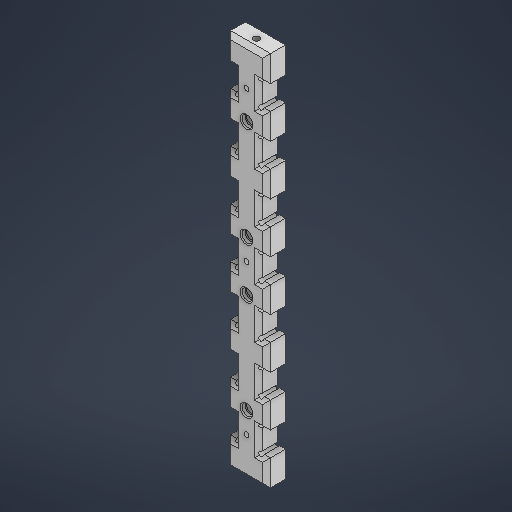
# Autodesk Inventor part: Locating_bar_V2_fit0
Saved by Autodesk Inventor 2026.1 (Build 301233020, 233B)
## iProperties
Created: 2023-09-05
Part Number: Locating_bar_V2_fit0
Material: Generic
Document SubType Name: Modeling
Designer: Joshua Harper
Density: 1 g/cm^3
Appearance: Default
Author: Joshua Harper
Autodesk Inventor part; units mm, degrees
ref_plane "YZ Plane" through (0, 0, 0) normal (1, 0, 0) x (0, 1, 0)
ref_plane "XZ Plane" through (0, 0, 0) normal (0, 1, 0) x (-1, 0, 0)
ref_plane "XY Plane" through (0, 0, 0) normal (0, 0, 1) x (1, 0, 0)
sketch "Sketch1" plane through (0, 0, 0) normal (0, 0, 1) x (1, 0, 0)
  line L0 (0, 94) -> (10, 94)
  line L1 (10, 94) -> (10, 81)
  line L2 (10, 81) -> (6, 81)
  line L3 (6, 81) -> (6, 69)
  line L4 (6, 69) -> (10, 69)
  line L5 (10, 69) -> (10, 56)
  line L6 (10, 56) -> (6, 56)
  line L7 (6, 56) -> (6, 44)
  line L8 (6, 44) -> (10, 44)
  line L9 (10, 44) -> (10, 31)
  line L10 (10, 31) -> (6, 31)
  line L11 (6, 31) -> (6, 19)
  line L12 (6, 19) -> (10, 19)
  line L13 (10, 19) -> (10, 6)
  line L14 (10, 6) -> (6, 6)
  line L15 (6, 6) -> (6, 0)
  line L16 (0, 0) -> (0, 65.9305) construction
  line L17 (0, 0) -> (38.6364, 0) construction
  line L18 (0, 94) -> (-10, 94)
  line L19 (-10, 94) -> (-10, 81)
  line L20 (-10, 81) -> (-6, 81)
  line L21 (-6, 81) -> (-6, 69)
  line L22 (-6, 69) -> (-10, 69)
  line L23 (-10, 69) -> (-10, 56)
  line L24 (-10, 56) -> (-6, 56)
  line L25 (-6, 56) -> (-6, 44)
  line L26 (-6, 44) -> (-10, 44)
  line L27 (-10, 44) -> (-10, 31)
  line L28 (-10, 31) -> (-6, 31)
  line L29 (-6, 31) -> (-6, 19)
  line L30 (-6, 19) -> (-10, 19)
  line L31 (-10, 19) -> (-10, 6)
  line L32 (-10, 6) -> (-6, 6)
  line L33 (-6, 6) -> (-6, 0)
  line L34 (0, 0) -> (-38.6364, 0) construction
  line L35 (0, -94) -> (10, -94)
  line L36 (10, -94) -> (10, -81)
  line L37 (10, -81) -> (6, -81)
  line L38 (6, -81) -> (6, -69)
  line L39 (6, -69) -> (10, -69)
  line L40 (10, -69) -> (10, -56)
  line L41 (10, -56) -> (6, -56)
  line L42 (6, -56) -> (6, -44)
  line L43 (6, -44) -> (10, -44)
  line L44 (10, -44) -> (10, -31)
  line L45 (10, -31) -> (6, -31)
  line L46 (6, -31) -> (6, -19)
  line L47 (6, -19) -> (10, -19)
  line L48 (10, -19) -> (10, -6)
  line L49 (10, -6) -> (6, -6)
  line L50 (6, -6) -> (6, 0)
  line L51 (0, 0) -> (0, -65.9305) construction
  line L52 (0, -94) -> (-10, -94)
  line L53 (-10, -94) -> (-10, -81)
  line L54 (-6, -69) -> (-10, -69)
  line L55 (-10, -81) -> (-6, -81)
  line L56 (-6, -81) -> (-6, -69)
  line L57 (-10, -69) -> (-10, -56)
  line L58 (-10, -56) -> (-6, -56)
  line L59 (-6, -56) -> (-6, -44)
  line L60 (-6, -44) -> (-10, -44)
  line L61 (-10, -44) -> (-10, -31)
  line L62 (-10, -31) -> (-6, -31)
  line L63 (-6, -31) -> (-6, -19)
  line L64 (-6, -19) -> (-10, -19)
  line L65 (-10, -19) -> (-10, -6)
  line L66 (-10, -6) -> (-6, -6)
  line L67 (-6, -6) -> (-6, 0)
  point P0 (6, 75)
  point P1 (5, 94)
  point P2 (-6, 75)
  point P3 (-5, 94)
  point P4 (6, -75)
  point P5 (5, -94)
  point P6 (-6, -75)
  point P7 (-5, -94)
  dimension "d0" = 10
  dimension "d1" = 13
  dimension "d2" = 12
  dimension "d3" = 6
  dimension "d4" = 6
  constraints: 136 end point, 55 symmetric about line, 44 point on line, 10 perpendicular, 6 collinear, 3 horizontal, 2 midpoint, 1 vertical
  measures "d0" distance of L0.start L0.end
  measures "d1" distance of L0.end L1.end
  measures "d2" distance between parallel lines of L4 L2
  measures "d3" distance from line of L16 point (6, 75)
  measures "d4" distance between parallel lines of L17 L14
extrude "Extrusion1" add sketch "Sketch1" along normal blind 9.5
chamfer "Chamfer1" distance 2 angle 45 64 edges at (-10, 87.5, 9.5) (10, 87.5, 9.5) (-8, 81, 9.5) (8, 81, 9.5) (6, 75, 9.5) (-6, 75, 9.5) (-8, 69, 9.5) (-10, 62.5, 9.5) (8, 69, 9.5) (10, 62.5, 9.5) (8, 56, 9.5) (-8, 56, 9.5) (6, 50, 9.5) (-6, 50, 9.5) (-8, 44, 9.5) (8, 44, 9.5) (10, 37.5, 9.5) (-10, 37.5, 9.5) (-8, 31, 9.5) (8, 31, 9.5) (6, 25, 9.5) (-6, 25, 9.5) (-8, 19, 9.5) (8, 19, 9.5) (10, 12.5, 9.5) (-10, 12.5, 9.5) (8, 6, 9.5) (-8, 6, 9.5) (-6, -3, 9.5) (-6, 3, 9.5) (6, 3, 9.5) (6, -3, 9.5) (8, -6, 9.5) (-8, -6, 9.5) (-10, -12.5, 9.5) (10, -12.5, 9.5) (8, -19, 9.5) (-8, -19, 9.5) (-6, -25, 9.5) (6, -25, 9.5) (8, -31, 9.5) (-8, -31, 9.5) (-10, -37.5, 9.5) (10, -37.5, 9.5) (-8, -44, 9.5) (8, -44, 9.5) (6, -50, 9.5) (-6, -50, 9.5) (-8, -56, 9.5) (8, -56, 9.5) (10, -62.5, 9.5) (-10, -62.5, 9.5) (8, -69, 9.5) (-8, -69, 9.5) (-6, -75, 9.5) (6, -75, 9.5) (8, -81, 9.5) (-8, -81, 9.5) (-10, -87.5, 9.5) (10, -87.5, 9.5) (5, -94, 9.5) (-5, -94, 9.5) (-5, 94, 9.5) (5, 94, 9.5)
sketch "Sketch2" plane through (-10, 94, 0) normal (0, 1, 0) x (1, 0, 0)
  line L0 (20, 0) -> (0, 0) projected
  line L1 (10, 0) -> (10, -4.5) construction
  line L2 (2, -9.5) -> (18, -9.5) projected
  dimension "d19" = 5
  constraints: 2 end point, 1 vertical
  measures "d19" distance from line of L2 L1.end
hole "Hole1" at (0, 94, 4.5) direction (0, -1, 0) diameter 3.242 depth 11.8 tip angle 118 thread size "M4x0.7" class "6H" standard "ANSI Metric M Profile"
mirror "Mirror1" about plane through (0, 0, 0) normal (0, 1, 0) of "Hole1"
sketch "Sketch3" plane through (0, 0, 0) normal (0, 0, -1) x (-1, 0, 0)
  line L0 (0, 0) -> (0, 75) construction
  line L1 (0, 0) -> (31.7018, 0) construction
  point P0 (0, -75)
  dimension "d28" = 75
  constraints: 4 end point, 1 coincident, 1 horizontal, 1 symmetric about line, 1 vertical
  measures "d28" distance of L0.end point (0, 0)
hole "Hole2" at (0, 0, 0) at (0, 75, 0) at (0, -75, 0) direction (0, 0, 1) diameter 2.459 end through all counterbore diameter 4 counterbore depth 2 thread size "M3x0.5" class "6H" standard "ANSI Metric M Profile"
sketch "Sketch4" plane through (0, 0, 0) normal (0, 0, -1) x (-1, 0, 0)
  circle A0 centre (0, 0) radius 1.2295 construction
  line L0 (0, 0) -> (0, -14.5) construction
  line L1 (15.0532, -2) -> (-13.6223, -2) construction
  point P0 (0, -64.5)
  point P1 (0, 10.5)
  point P2 (0, 60.5)
  dimension "d36" = 14.5
  dimension "d82" = 64.5
  dimension "d83" = 2
  constraints: 4 end point, 2 symmetric about line, 1 horizontal, 1 vertical
  measures "d36" distance of L0.end point (0, 0)
  measures "d82" distance of point (0, -64.5) point (0, 0)
  measures "d83" distance from line of L1 point (0, 0)
hole "Hole3" at (0, -14.5, 0) at (0, -64.5, 0) at (0, 10.5, 0) at (0, 60.5, 0) direction (0, 0, 1) diameter 4.5 end through all counterbore diameter 8 counterbore depth 3 clearance for "Slotted Cheese Head Screw DIN 84" size "M4" standard "DIN"
sketch "Sketch5" plane through (0, 0, 9.5) normal (0, 0, 1) x (1, 0, 0)
  line L0 (-10, -81) -> (-10, -94) construction
  line L1 (-10, -94) -> (10, -94) construction
  circle A0 centre (0, -14.5) radius 2.25 construction
  circle A1 centre (0, -14.5) radius 2.25 construction
  circle A2 centre (0, -64.5) radius 2.25 construction
  circle A3 centre (0, -64.5) radius 2.25 construction
  circle A4 centre (0, 0) radius 1.2295 construction
  circle A5 centre (0, 10.5) radius 2.25 construction
  circle A6 centre (0, 10.5) radius 2.25 construction
  circle A7 centre (0, 60.5) radius 2.25 construction
  circle A8 centre (0, 60.5) radius 2.25 construction
  circle A9 centre (0, 10.5) radius 2.25 projected
  circle A10 centre (0, 60.5) radius 2.25 projected
  constraints: 6 centre point, 6 coincident, 5 concentric, 1 vertical alignment
hole "Hole4" at (0, -64.5, 9.5) at (0, -14.5, 9.5) at (0, 60.5, 9.5) at (0, 10.5, 9.5) direction (0, 0, -1) diameter 5.5 depth 2 tip angle 118
chamfer "Chamfer2" distance 0.5 angle 45 4 edges at (0, -61.75, 9.5) (0, -11.75, 9.5) (0, 13.25, 9.5) (0, 63.25, 9.5)
chamfer "Chamfer3" distance 0.5 angle 45 3 edges at (0, -2, 0) (0, 73, 0) (0, -77, 0)
sketch "Sketch6" plane through (0, 0, 0) normal (0, 0, -1) x (-1, 0, 0)
  circle A0 centre (6, 6) radius 1
  line L0 (0, 0) -> (11.6098, 0) construction
  line L1 (0, 0) -> (0, -13.3331) construction
  circle A1 centre (6, 19) radius 1
  circle A2 centre (6, 31) radius 1
  circle A3 centre (6, 44) radius 1
  circle A4 centre (6, 56) radius 1
  circle A5 centre (6, 69) radius 1
  circle A6 centre (6, 81) radius 1
  circle A7 centre (6, -6) radius 1
  circle A8 centre (6, -19) radius 1
  circle A9 centre (6, -31) radius 1
  circle A10 centre (6, -44) radius 1
  circle A11 centre (6, -56) radius 1
  circle A12 centre (6, -69) radius 1
  circle A13 centre (6, -81) radius 1
  circle A14 centre (-6, 6) radius 1
  circle A15 centre (-6, 19) radius 1
  circle A16 centre (-6, 31) radius 1
  circle A17 centre (-6, 44) radius 1
  circle A18 centre (-6, 56) radius 1
  circle A19 centre (-6, 69) radius 1
  circle A20 centre (-6, 81) radius 1
  circle A21 centre (-6, -6) radius 1
  circle A22 centre (-6, -19) radius 1
  circle A23 centre (-6, -31) radius 1
  circle A24 centre (-6, -44) radius 1
  circle A25 centre (-6, -56) radius 1
  circle A26 centre (-6, -69) radius 1
  circle A27 centre (-6, -81) radius 1
  point P0 (4, 67)
  dimension "d64" = 2
  constraints: 28 centre point, 24 symmetric about line, 6 equal radius, 4 coincident, 4 end point, 1 horizontal, 1 vertical, 21 other
  measures "d64" diameter of A0
extrude "Extrusion2" cut sketch "Sketch6" against normal through all
equation "\"d1\" = r_space"
equation "\"r_space\" = 13"
body "Solid1"
